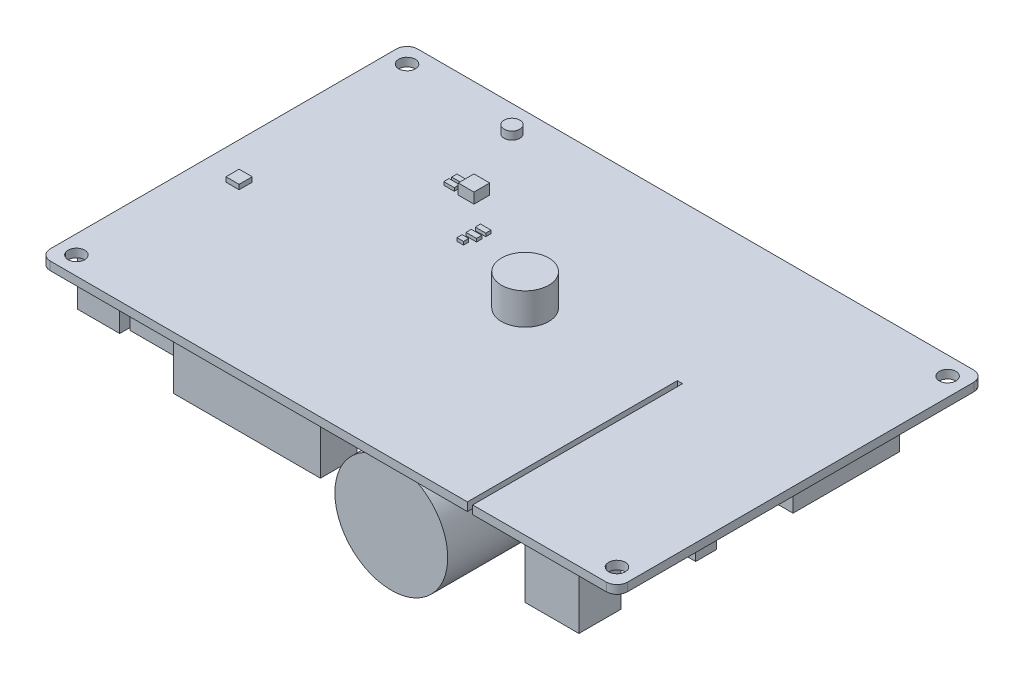
GridUp-PCB (Autodesk Fusion 360 design; units mm, degrees)
part number: 2026-09-14-08-15-55-205
Autodesk Fusion 360 part; units mm, degrees
sketch "Çizim1" plane through (0, 0, 0) normal (0, 0, 1) x (1, 0, 0)
  line L0 (0, 0) -> (110, 0)
  line L1 (110, 0) -> (110, 70)
  line L2 (110, 70) -> (0, 70)
  line L3 (0, 70) -> (0, 0)
extrude "Ekstrüzyon1" add sketch "Çizim1" along normal blind 1.6 makes body 1
fillet "Radyus1" radius 2 4 edges at (0, 70, 0.8) (110, 70, 0.8) (110, 0, 0.8) (0, 0, 0.8) on bodies 1
sketch "Çizim2" plane through (0, 0, 0) normal (0, 0, 1) x (1, 0, 0)
  circle A0 centre (3.5, 3.5) radius 1.6
  circle A1 centre (106.5, 3.5) radius 1.6
  circle A2 centre (3.5, 66.5) radius 1.6
  circle A3 centre (106.5, 66.5) radius 1.6
  line L0 (81.5, -1) -> (82.5, -1)
  line L1 (82.5, -1) -> (82.5, 40)
  line L2 (82.5, 40) -> (81.5, 40)
  line L3 (81.5, 40) -> (81.5, -1)
extrude "Ekstrüzyon2" cut sketch "Çizim2" along normal mid plane 10 bodies 1
ref_plane "WorkPlane1" through (0, 0, 1.6) normal (0, 0, 1) x (1, 0, 0)
sketch "Çizim3" plane through (0, 0, 1.6) normal (0, 0, 1) x (1, 0, 0)
  circle A0 centre (55, 37.5) radius 4.5
extrude "Ekstrüzyon3" add sketch "Çizim3" along normal blind 6 separate body makes body 2
ref_plane "WorkPlane2" through (0, 0, 1.6) normal (0, 0, 1) x (1, 0, 0)
sketch "Çizim4" plane through (0, 0, 1.6) normal (0, 0, 1) x (1, 0, 0)
  line L0 (5.75, 29.75) -> (8.25, 29.75)
  line L1 (8.25, 29.75) -> (8.25, 32.25)
  line L2 (8.25, 32.25) -> (5.75, 32.25)
  line L3 (5.75, 32.25) -> (5.75, 29.75)
extrude "Ekstrüzyon4" add sketch "Çizim4" along normal blind 0.9 separate body makes body 3
ref_plane "WorkPlane3" through (0, 0, 1.6) normal (0, 0, 1) x (1, 0, 0)
sketch "Çizim5" plane through (0, 0, 1.6) normal (0, 0, 1) x (1, 0, 0)
  circle A0 centre (25, 65) radius 1.5
extrude "Ekstrüzyon5" add sketch "Çizim5" along normal blind 1.5 separate body makes body 4
ref_plane "WorkPlane4" through (0, 0, 1.6) normal (0, 0, 1) x (1, 0, 0)
sketch "Çizim6" plane through (0, 0, 1.6) normal (0, 0, 1) x (1, 0, 0)
  line L0 (37.5, 45.5) -> (39.5, 45.5)
  line L1 (39.5, 45.5) -> (39.5, 46.5)
  line L2 (39.5, 46.5) -> (37.5, 46.5)
  line L3 (37.5, 46.5) -> (37.5, 45.5)
extrude "Ekstrüzyon6" add sketch "Çizim6" along normal blind 0.6 separate body makes body 5
ref_plane "WorkPlane5" through (0, 0, 1.6) normal (0, 0, 1) x (1, 0, 0)
sketch "Çizim7" plane through (0, 0, 1.6) normal (0, 0, 1) x (1, 0, 0)
  line L0 (37.5, 43.75) -> (39.5, 43.75)
  line L1 (39.5, 43.75) -> (39.5, 44.75)
  line L2 (39.5, 44.75) -> (37.5, 44.75)
  line L3 (37.5, 44.75) -> (37.5, 43.75)
extrude "Ekstrüzyon7" add sketch "Çizim7" along normal blind 0.6 separate body makes body 6
ref_plane "WorkPlane6" through (0, 0, 1.6) normal (0, 0, 1) x (1, 0, 0)
sketch "Çizim8" plane through (0, 0, 1.6) normal (0, 0, 1) x (1, 0, 0)
  line L0 (37.5, 42) -> (38.75, 42)
  line L1 (38.75, 42) -> (38.75, 43)
  line L2 (38.75, 43) -> (37.5, 43)
  line L3 (37.5, 43) -> (37.5, 42)
extrude "Ekstrüzyon8" add sketch "Çizim8" along normal blind 0.6 separate body makes body 7
ref_plane "WorkPlane7" through (0, 0, 1.6) normal (0, 0, 1) x (1, 0, 0)
sketch "Çizim9" plane through (0, 0, 1.6) normal (0, 0, 1) x (1, 0, 0)
  line L0 (27, 51.5) -> (29, 51.5)
  line L1 (29, 51.5) -> (29, 52.5)
  line L2 (29, 52.5) -> (27, 52.5)
  line L3 (27, 52.5) -> (27, 51.5)
extrude "Ekstrüzyon9" add sketch "Çizim9" along normal blind 0.6 separate body makes body 8
ref_plane "WorkPlane8" through (0, 0, 1.6) normal (0, 0, 1) x (1, 0, 0)
sketch "Çizim10" plane through (0, 0, 1.6) normal (0, 0, 1) x (1, 0, 0)
  line L0 (27, 50) -> (29, 50)
  line L1 (29, 50) -> (29, 51)
  line L2 (29, 51) -> (27, 51)
  line L3 (27, 51) -> (27, 50)
extrude "Ekstrüzyon10" add sketch "Çizim10" along normal blind 0.6 separate body makes body 9
ref_plane "WorkPlane9" through (0, 0, 1.6) normal (0, 0, 1) x (1, 0, 0)
sketch "Çizim11" plane through (0, 0, 1.6) normal (0, 0, 1) x (1, 0, 0)
  line L0 (30, 49.75) -> (33, 49.75)
  line L1 (33, 49.75) -> (33, 52.75)
  line L2 (33, 52.75) -> (30, 52.75)
  line L3 (30, 52.75) -> (30, 49.75)
extrude "Ekstrüzyon11" add sketch "Çizim11" along normal blind 2 separate body makes body 10
ref_plane "WorkPlane10" through (0, 0, 0) normal (0, 0, 1) x (1, 0, 0)
sketch "Çizim12" plane through (0, 0, 0) normal (0, 0, 1) x (1, 0, 0)
  line L0 (6, 44.8) -> (24, 44.8)
  line L1 (24, 44.8) -> (24, 64)
  line L2 (24, 64) -> (6, 64)
  line L3 (6, 64) -> (6, 44.8)
extrude "Ekstrüzyon12" add sketch "Çizim12" against normal blind 3.2 separate body makes body 11
ref_plane "WorkPlane11" through (0, 0, 0) normal (0, 0, 1) x (1, 0, 0)
sketch "Çizim13" plane through (0, 0, 0) normal (0, 0, 1) x (1, 0, 0)
  line L0 (66, 43.75) -> (99.8, 43.75)
  line L1 (99.8, 43.75) -> (99.8, 64.05)
  line L2 (99.8, 64.05) -> (66, 64.05)
  line L3 (66, 64.05) -> (66, 43.75)
extrude "Ekstrüzyon13" add sketch "Çizim13" against normal blind 13 separate body makes body 12
ref_plane "WorkPlane12" through (0, 0, 0) normal (0, 0, 1) x (1, 0, 0)
sketch "Çizim14" plane through (0, 0, 0) normal (0, 0, 1) x (1, 0, 0)
  line L0 (88, 22.25) -> (94.1, 22.25)
  line L1 (94.1, 22.25) -> (94.1, 25)
  line L2 (94.1, 25) -> (88, 25)
  line L3 (88, 25) -> (88, 22.25)
extrude "Ekstrüzyon14" add sketch "Çizim14" against normal blind 2.6 separate body makes body 13
ref_plane "WorkPlane13" through (0, 0, 0) normal (0, 0, 1) x (1, 0, 0)
sketch "Çizim15" plane through (0, 0, 0) normal (0, 0, 1) x (1, 0, 0)
  line L0 (96.5, 21.5) -> (103.5, 21.5)
  line L1 (103.5, 21.5) -> (103.5, 25.5)
  line L2 (103.5, 25.5) -> (96.5, 25.5)
  line L3 (96.5, 25.5) -> (96.5, 21.5)
extrude "Ekstrüzyon15" add sketch "Çizim15" against normal blind 8 separate body makes body 14
ref_plane "WorkPlane14" through (0, 0, 0) normal (0, 0, 1) x (1, 0, 0)
sketch "Çizim16" plane through (0, 0, 0) normal (0, 0, 1) x (1, 0, 0)
  line L0 (92, 0.5) -> (102.25, 0.5)
  line L1 (102.25, 0.5) -> (102.25, 8.5)
  line L2 (102.25, 8.5) -> (92, 8.5)
  line L3 (92, 8.5) -> (92, 0.5)
extrude "Ekstrüzyon16" add sketch "Çizim16" against normal blind 10 separate body makes body 15
ref_plane "WorkPlane15" through (0, 0, 0) normal (0, 0, 1) x (1, 0, 0)
sketch "Çizim17" plane through (0, 0, 0) normal (0, 0, 1) x (1, 0, 0)
  line L0 (70, 35) -> (76.5, 35)
  line L1 (76.5, 35) -> (76.5, 42)
  line L2 (76.5, 42) -> (70, 42)
  line L3 (70, 42) -> (70, 35)
extrude "Ekstrüzyon17" add sketch "Çizim17" against normal blind 1.7 separate body makes body 16
ref_plane "WorkPlane16" through (0, 0, 0) normal (0, 0, 1) x (1, 0, 0)
sketch "Çizim18" plane through (0, 0, 0) normal (0, 0, 1) x (1, 0, 0)
  line L0 (76.75, 39.1) -> (81, 39.1)
  line L1 (81, 39.1) -> (81, 41.75)
  line L2 (81, 41.75) -> (76.75, 41.75)
  line L3 (76.75, 41.75) -> (76.75, 39.1)
extrude "Ekstrüzyon18" add sketch "Çizim18" against normal blind 1.5 separate body makes body 17
ref_plane "WorkPlane17" through (0, 0, 0) normal (0, 0, 1) x (1, 0, 0)
sketch "Çizim19" plane through (0, 0, 0) normal (0, 0, 1) x (1, 0, 0)
  line L0 (76.75, 35.1) -> (81, 35.1)
  line L1 (81, 35.1) -> (81, 37.75)
  line L2 (81, 37.75) -> (76.75, 37.75)
  line L3 (76.75, 37.75) -> (76.75, 35.1)
extrude "Ekstrüzyon19" add sketch "Çizim19" against normal blind 1.5 separate body makes body 18
ref_plane "WorkPlane18" through (0, 0, 0) normal (0, 0, 1) x (1, 0, 0)
sketch "Çizim20" plane through (0, 0, 0) normal (0, 0, 1) x (1, 0, 0)
  line L0 (75, 44.5) -> (77, 44.5)
  line L1 (77, 44.5) -> (77, 45.5)
  line L2 (77, 45.5) -> (75, 45.5)
  line L3 (75, 45.5) -> (75, 44.5)
extrude "Ekstrüzyon20" add sketch "Çizim20" against normal blind 0.6 separate body makes body 19
ref_plane "WorkPlane19" through (0, 0, 0) normal (0, 0, 1) x (1, 0, 0)
sketch "Çizim21" plane through (0, 0, 0) normal (0, 0, 1) x (1, 0, 0)
  line L0 (75, 29.5) -> (77, 29.5)
  line L1 (77, 29.5) -> (77, 30.5)
  line L2 (77, 30.5) -> (75, 30.5)
  line L3 (75, 30.5) -> (75, 29.5)
extrude "Ekstrüzyon21" add sketch "Çizim21" against normal blind 0.6 separate body makes body 20
ref_plane "WorkPlane20" through (0, 0, 0) normal (0, 0, 1) x (1, 0, 0)
sketch "Çizim22" plane through (0, 0, 0) normal (0, 0, 1) x (1, 0, 0)
  line L0 (75, 28) -> (77, 28)
  line L1 (77, 28) -> (77, 29)
  line L2 (77, 29) -> (75, 29)
  line L3 (75, 29) -> (75, 28)
extrude "Ekstrüzyon22" add sketch "Çizim22" against normal blind 0.6 separate body makes body 21
ref_plane "WorkPlane21" through (0, 13.75, 0) normal (0, 1, 0) x (0, 0, 1)
sketch "Çizim23" plane through (0, 13.75, 0) normal (0, 1, 0) x (1, 0, 0)
  circle A0 centre (65.75, 10.75) radius 10.75
extrude "Ekstrüzyon23" add sketch "Çizim23" along normal mid plane 25 separate body makes body 22
ref_plane "WorkPlane22" through (0, 0, 0) normal (0, 0, 1) x (1, 0, 0)
sketch "Çizim24" plane through (0, 0, 0) normal (0, 0, 1) x (1, 0, 0)
  line L0 (41.25, 14) -> (46.25, 14)
  line L1 (46.25, 14) -> (46.25, 20)
  line L2 (46.25, 20) -> (41.25, 20)
  line L3 (41.25, 20) -> (41.25, 14)
extrude "Ekstrüzyon24" add sketch "Çizim24" against normal blind 1.5 separate body makes body 23
ref_plane "WorkPlane23" through (0, 0, 0) normal (0, 0, 1) x (1, 0, 0)
sketch "Çizim25" plane through (0, 0, 0) normal (0, 0, 1) x (1, 0, 0)
  line L0 (47.5, 15) -> (48.5, 15)
  line L1 (48.5, 15) -> (48.5, 17)
  line L2 (48.5, 17) -> (47.5, 17)
  line L3 (47.5, 17) -> (47.5, 15)
extrude "Ekstrüzyon25" add sketch "Çizim25" against normal blind 0.6 separate body makes body 24
ref_plane "WorkPlane24" through (0, 0, 0) normal (0, 0, 1) x (1, 0, 0)
sketch "Çizim26" plane through (0, 0, 0) normal (0, 0, 1) x (1, 0, 0)
  line L0 (1, 6.25) -> (9, 6.25)
  line L1 (9, 6.25) -> (9, 21.5)
  line L2 (9, 21.5) -> (1, 21.5)
  line L3 (1, 21.5) -> (1, 6.25)
extrude "Ekstrüzyon26" add sketch "Çizim26" against normal blind 10 separate body makes body 25
ref_plane "WorkPlane25" through (0, 0, 0) normal (0, 0, 1) x (1, 0, 0)
sketch "Çizim27" plane through (0, 0, 0) normal (0, 0, 1) x (1, 0, 0)
  line L0 (25, 14) -> (27, 14)
  line L1 (27, 14) -> (27, 15)
  line L2 (27, 15) -> (25, 15)
  line L3 (25, 15) -> (25, 14)
extrude "Ekstrüzyon27" add sketch "Çizim27" against normal blind 0.6 separate body makes body 26
ref_plane "WorkPlane26" through (0, 0, 0) normal (0, 0, 1) x (1, 0, 0)
sketch "Çizim28" plane through (0, 0, 0) normal (0, 0, 1) x (1, 0, 0)
  line L0 (28, 14) -> (30, 14)
  line L1 (30, 14) -> (30, 15)
  line L2 (30, 15) -> (28, 15)
  line L3 (28, 15) -> (28, 14)
extrude "Ekstrüzyon28" add sketch "Çizim28" against normal blind 0.6 separate body makes body 27
ref_plane "WorkPlane27" through (0, 0, 0) normal (0, 0, 1) x (1, 0, 0)
sketch "Çizim29" plane through (0, 0, 0) normal (0, 0, 1) x (1, 0, 0)
  line L0 (31, 14) -> (33, 14)
  line L1 (33, 14) -> (33, 15)
  line L2 (33, 15) -> (31, 15)
  line L3 (31, 15) -> (31, 14)
extrude "Ekstrüzyon29" add sketch "Çizim29" against normal blind 0.6 separate body makes body 28
ref_plane "WorkPlane28" through (0, 0, 0) normal (0, 0, 1) x (1, 0, 0)
sketch "Çizim30" plane through (0, 0, 0) normal (0, 0, 1) x (1, 0, 0)
  line L0 (34, 14) -> (36, 14)
  line L1 (36, 14) -> (36, 15)
  line L2 (36, 15) -> (34, 15)
  line L3 (34, 15) -> (34, 14)
extrude "Ekstrüzyon30" add sketch "Çizim30" against normal blind 0.6 separate body makes body 29
ref_plane "WorkPlane29" through (0, 0, 0) normal (0, 0, 1) x (1, 0, 0)
sketch "Çizim31" plane through (0, 0, 0) normal (0, 0, 1) x (1, 0, 0)
  line L0 (37, 13) -> (39, 13)
  line L1 (39, 13) -> (39, 15)
  line L2 (39, 15) -> (37, 15)
  line L3 (37, 15) -> (37, 13)
extrude "Ekstrüzyon31" add sketch "Çizim31" against normal blind 0.6 separate body makes body 30
ref_plane "WorkPlane30" through (0, 0, 0) normal (0, 0, 1) x (1, 0, 0)
sketch "Çizim32" plane through (0, 0, 0) normal (0, 0, 1) x (1, 0, 0)
  line L0 (25, 0.5) -> (53, 0.5)
  line L1 (53, 0.5) -> (53, 7.5)
  line L2 (53, 7.5) -> (25, 7.5)
  line L3 (25, 7.5) -> (25, 0.5)
extrude "Ekstrüzyon32" add sketch "Çizim32" against normal blind 9 separate body makes body 31
ref_plane "WorkPlane31" through (0, 0, 0) normal (0, 0, 1) x (1, 0, 0)
sketch "Çizim33" plane through (0, 0, 0) normal (0, 0, 1) x (1, 0, 0)
  line L0 (11, 6.25) -> (24, 6.25)
  line L1 (24, 6.25) -> (24, 11.25)
  line L2 (24, 11.25) -> (11, 11.25)
  line L3 (11, 11.25) -> (11, 6.25)
extrude "Ekstrüzyon33" add sketch "Çizim33" against normal blind 8.5 separate body makes body 32
equation "d45 = -( 3.2 mm )"
equation "d49 = -( 13 mm )"
equation "d53 = -( 2.6 mm )"
equation "d57 = -( 8 mm )"
equation "d61 = -( 10 mm )"
equation "d65 = -( 1.7 mm )"
equation "d69 = -( 1.5 mm )"
equation "d73 = -( 1.5 mm )"
equation "d77 = -( 0.6 mm )"
equation "d81 = -( 0.6 mm )"
equation "d85 = -( 0.6 mm )"
equation "d93 = -( 1.5 mm )"
equation "d97 = -( 0.6 mm )"
equation "d101 = -( 10 mm )"
equation "d105 = -( 0.6 mm )"
equation "d109 = -( 0.6 mm )"
equation "d113 = -( 0.6 mm )"
equation "d117 = -( 0.6 mm )"
equation "d121 = -( 0.6 mm )"
equation "d125 = -( 9 mm )"
equation "d129 = -( 8.5 mm )"
named bodies: "PCB", "MLX90640", "SHT31", "LED", "R_pullup1", "R_pullup2", "C_100n", "EN_RC1", "EN_RC2", "Reset", "ESP32-S3-WROOM-1U", "RAC05-05SK", "F1", "MOV", "Klemens 230V", "LDO SOT-223", "D1", "D2", "R_sarj", "Bolucu1", "Bolucu2", "Superkap", "MAX3485", "R120", "Klemens RS-485", "R_burden1", "R_burden2", "R_burden3", "R_burden4", "R_bias", "Klemens CT", "Genisleme 2x5"
